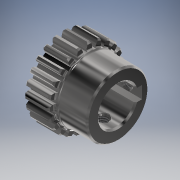
# Autodesk Inventor part: 歯車m1,z23
Saved by Autodesk Inventor 2019.2 (Build 232265000, 265)
## iProperties
Category: PARTsolutions
Company: KHK
Created: 2018-12-15
Part Number: 歯車m1,z23
Material: 鋼、高強度、低合金
Catalog Web Link: www.cadenas.de
Description: Ground Spur Gears (SSG)-
Vendor: KHK
Document SubType Name: Modeling
Designer: psadmin
Manufacturer: KHK
Mass: 4.81881 g
Surface Area: 26.6249 cm^2
Volume: 4.81881 cm^3
Density: 7.85 g/cm^3
Appearance: 鋼 - つや出し
PSOL_IDENT_0: {$CADENAS_DATA\23d-libs\khk\spur_gears\ground_spur_gears_ssg.prj},180 {VTYP=3D},{NB=SSG1-23J12},{LIN
PSOL_IDENT_1: A=SSG1-23J12},{NN=Ground Spur Gears (SSG)},{DATE=17.03.2017 04:28:20},{GEOMDATE=10.12.2014 11:17:00}
PSOL_IDENT_2: ,{VERSION=},{LINEID=18740},{WBVAR=},{WBNUMERIC=}  {NB=SSG1-23J12},{LINA=SSG1-23J12},{KT=DUMMY},{CN=S
PSOL_IDENT_3: SG1-23J12},{M=1.0},{Z=23},{A=12},{B=20},{C=23.0},{D=25.0},{E=8},{F=10},{G=18},{H=0},{I=0},{K=4},{KD=
PSOL_IDENT_4: 1.8},{M1=M4},{J=5.0},{S=S1K},{R=0.5},{N=0.5},{L=0.5},{L2=0.5},{X=3},{M11=4},{XX=4},{HIDE=0},{CBD1=0.
PSOL_IDENT_5: 0},{CBD2=0.0}
NN: Ground Spur Gears (SSG)
NB: SSG1-23J12
NBSYN: $CN.
LINA: SSG1-23J12
CN: SSG1-23J12
M: 1
Z: 23
A: 12
B: 20
C: 23
D: 25
E: 8
F: 10
G: 18
H: 0
I: 0
K: 4
KD: 1.8
M1: M4
J: 5
S: S1K
SUPPLIER: KHK
ARTICLENO: SSG1-23J12
BOMINFO: SSG1-23J12
CREATOR: CADENAS GmbH
Title: SSG1-23J12
Author: Cadenas PARTsolutions
Autodesk Inventor part; units mm, degrees
ref_plane "YZ Plane" through (0, 0, 0) normal (1, 0, 0) x (0, 1, 0)
ref_plane "XZ Plane" through (0, 0, 0) normal (0, 1, 0) x (-1, 0, 0)
ref_plane "XY Plane" through (0, 0, 0) normal (0, 0, 1) x (1, 0, 0)
sketch "Sketch_1" plane through (0, 0, 0) normal (0, 0, 1) x (1, 0, 0)
  line L0 (18, 0) -> (0, 0)
  line L1 (0, 6.5) -> (0.5, 6)
  line L2 (0.5, 6) -> (17.5, 6)
  line L3 (17.5, 6) -> (18, 6.5)
  line L4 (18, 6.5) -> (18, 9.5)
  line L5 (18, 9.5) -> (17.5, 10)
  line L6 (17.5, 10) -> (9, 10)
  arc A0 (8, 11) -> (9, 10) centre (9, 11) ccw
  line L7 (8, 11) -> (8, 12)
  line L8 (8, 12) -> (7.5, 12.5)
  line L9 (7.5, 12.5) -> (0.5, 12.5)
  line L10 (0.5, 12.5) -> (0, 12)
  line L11 (0, 12) -> (0, 6.5)
  constraints: 24 end point, 2 point on circle, 1 centre point
revolve "Revolution1" add sketch "Sketch_1" angle 360 about axis through (18, 0, 0) along (1, 0, 0)
sketch "Sketch_6" plane through (0, 0, 0) normal (1, 0, 0) x (0, 1, 0)
  line L0 (4.2, 2) -> (4.2, -2)
  line L1 (4.2, -2) -> (7.8, -2)
  line L2 (7.8, -2) -> (7.8, 2)
  line L3 (7.8, 2) -> (4.2, 2)
  constraints: 8 end point
extrude "Extrusion1" cut sketch "Sketch_6" along normal blind 20
sketch "Sketch_2" plane through (0, 0, 0) normal (0, 0, 1) x (1, 0, 0)
  line L0 (13, 0) -> (13, 12.5)
  line L1 (13, 12.5) -> (15, 12.5)
  line L2 (15, 12.5) -> (15, 10)
  line L3 (15, 10) -> (14.621, 9.621)
  line L4 (14.621, 9.621) -> (14.621, 8.179)
  line L5 (14.621, 8.179) -> (15, 7.8)
  line L6 (15, 7.8) -> (15, 0)
  line L7 (15, 0) -> (13, 0)
  line L8 (13, 0) -> (13, 12.5)
  constraints: 18 end point
revolve "Revolution2" cut sketch "Sketch_2" angle 360 about axis through (13, 0, 0) along (0, -1, 0)
thread "Thread1" size "M4x0.7" class "6H" standard "ISO Metric profile" full length
sketch "Sketch_5" plane through (0, 0, 0) normal (0, 1, 0) x (-1, 0, 0)
  line L0 (-13, 0) -> (-13, -12.5)
  line L1 (-13, -12.5) -> (-15, -12.5)
  line L2 (-15, -12.5) -> (-15, -10)
  line L3 (-15, -10) -> (-14.621, -9.621)
  line L4 (-14.621, -9.621) -> (-14.621, -6.379)
  line L5 (-14.621, -6.379) -> (-15, -6)
  line L6 (-15, -6) -> (-15, 0)
  line L7 (-15, 0) -> (-13, 0)
  line L8 (-13, 0) -> (-13, -12.5)
  constraints: 18 end point
revolve "Revolution3" cut sketch "Sketch_5" angle 360 about axis through (13, 0, 0) along (0, 0, 1)
thread "Thread2" size "M4x0.7" class "6H" standard "ISO Metric profile" full length
sketch "スケッチ5" plane through (0, 0, 0) normal (-1, 0, 0) x (0, 0, 1)
  arc A0 (0.6057, 10.9584) -> (0.5767, 10.7911) centre (1.6476, 10.6916) ccw
  arc A1 (0.7884, 11.4814) -> (0.6057, 10.9584) centre (3.4791, 10.2479) ccw
  arc A2 (1.3493, 12.427) -> (0.7884, 11.4814) centre (5.4528, 9.354) ccw
  arc A3 (-2.3733, 10.7154) -> (-2.3561, 10.5465) centre (-1.2981, 10.7397) ccw
  arc A4 (-2.3384, 11.2683) -> (-2.3733, 10.7154) centre (0.5852, 10.8065) ccw
  arc A5 (-2.0535, 12.3302) -> (-2.3384, 11.2683) centre (2.7269, 10.4783) ccw
  arc A6 (-5.1763, 9.6778) -> (-5.1141, 9.5197) centre (-4.1474, 9.9912) ccw
  arc A7 (-5.2919, 10.2196) -> (-5.1763, 9.6778) centre (-2.3521, 10.5636) ccw
  arc A8 (-5.304, 11.3189) -> (-5.2919, 10.2196) centre (-0.2013, 10.8254) ccw
  arc A9 (-7.5954, 7.9224) -> (-7.4929, 7.7869) centre (-6.6892, 8.5017) ccw
  arc A10 (-7.8529, 8.4129) -> (-7.5954, 7.9224) centre (-5.1149, 9.5373) ccw
  arc A11 (-8.1611, 9.4682) -> (-7.8529, 8.4129) centre (-3.1145, 10.3697) ccw
  arc A12 (-9.4511, 5.5794) -> (-9.3159, 5.4766) centre (-8.7349, 6.3817) ccw
  arc A13 (-9.8314, 5.9822) -> (-9.4511, 5.5794) centre (-7.4983, 7.8037) ccw
  arc A14 (-10.413, 6.9152) -> (-9.8314, 5.9822) centre (-5.7967, 9.1449) ccw
  arc A15 (-10.606, 2.8226) -> (-10.448, 2.7601) centre (-10.1328, 3.7884) ccw
  arc A16 (-11.0808, 3.1079) -> (-10.606, 2.8226) centre (-9.3257, 5.4913) ccw
  arc A17 (-11.8925, 3.8494) -> (-11.0808, 3.1079) centre (-8.049, 7.2418) ccw
  arc A18 (-10.9742, -0.1435) -> (-10.8053, -0.1611) centre (-10.7791, 0.9141) ccw
  arc A19 (-11.5084, 0.0031) -> (-10.9742, -0.1435) centre (-10.4614, 2.7716) ccw
  arc A20 (-12.4901, 0.4981) -> (-11.5084, 0.0031) centre (-9.7043, 4.8017) ccw
  arc A21 (-10.5285, -3.099) -> (-10.3611, -3.0703) centre (-10.626, -2.0279) ccw
  arc A22 (-11.0825, -3.102) -> (-10.5285, -3.099) centre (-10.8212, -0.1536) ccw
  arc A23 (-12.1613, -2.8902) -> (-11.0825, -3.102) centre (-10.6399, 2.0054) ccw
  arc A24 (-9.302, -5.8247) -> (-9.1485, -5.7519) centre (-9.6849, -4.8196) ccw
  arc A25 (-9.8346, -5.977) -> (-9.302, -5.8247) centre (-10.3785, -3.0675) ccw
  arc A26 (-10.9306, -6.0641) -> (-9.8346, -5.977) centre (-10.7864, -0.9395) ccw
  arc A27 (-7.3856, -8.1183) -> (-7.2575, -8.0068) centre (-8.0254, -7.2538) ccw
  arc A28 (-7.8574, -8.4087) -> (-7.3856, -8.1183) centre (-9.166, -5.7538) ccw
  arc A29 (-8.8892, -8.7882) -> (-7.8574, -8.4087) centre (-10.133, -3.8148) ccw
  arc A30 (-4.9214, -9.8098) -> (-4.8281, -9.6679) centre (-5.7707, -9.1501) ccw
  arc A31 (-5.2974, -10.2167) -> (-4.9214, -9.8098) centre (-7.2738, -8.0134) ccw
  arc A32 (-6.1885, -10.8606) -> (-5.2974, -10.2167) centre (-8.728, -6.4072) ccw
  arc A33 (-2.0922, -10.7738) -> (-2.0407, -10.612) centre (-3.0881, -10.3677) ccw
  arc A34 (-2.3445, -11.2671) -> (-2.0922, -10.7738) centre (-4.8421, -9.6787) ccw
  arc A35 (-3.0288, -12.1275) -> (-2.3445, -11.2671) centre (-6.6757, -8.5244) ccw
  arc A36 (0.8921, -10.9388) -> (0.8981, -10.7691) centre (-0.1764, -10.8164) ccw
  arc A37 (0.7823, -11.4818) -> (0.8921, -10.9388) centre (-2.0512, -10.6262) ccw
  arc A38 (0.3554, -12.4949) -> (0.7823, -11.4818) centre (-4.1283, -10.0094) ccw
  arc A39 (3.8103, -10.2925) -> (3.7702, -10.1274) centre (2.7483, -10.4629) ccw
  arc A40 (3.851, -10.845) -> (3.8103, -10.2925) centre (0.8917, -10.7855) ccw
  arc A41 (3.7133, -11.9357) -> (3.851, -10.845) centre (-1.2747, -10.752) ccw
  arc A42 (6.4459, -8.8828) -> (6.3628, -8.7347) centre (5.4693, -9.3334) ccw
  arc A43 (6.6342, -9.4038) -> (6.4459, -8.8828) centre (3.7686, -10.145) ccw
  arc A44 (6.7959, -10.4912) -> (6.6342, -9.4038) centre (1.6734, -10.6972) ccw
  arc A45 (8.6034, -6.8143) -> (8.4834, -6.6941) centre (7.7846, -7.5117) ccw
  arc A46 (8.9253, -7.2652) -> (8.6034, -6.8143) centre (6.3659, -8.752) ccw
  arc A47 (9.3744, -8.2687) -> (8.9253, -7.2652) centre (4.4975, -9.849) ccw
  arc A48 (10.1228, -4.2405) -> (9.9749, -4.1571) centre (9.5225, -5.1329) ccw
  arc A49 (10.5544, -4.5878) -> (10.1228, -4.2405) centre (8.4911, -6.71) ccw
  arc A50 (11.2576, -5.4329) -> (10.5544, -4.5878) centre (6.9879, -8.2704) ccw
  arc A51 (10.8915, -1.3521) -> (10.7266, -1.3118) centre (10.5542, -2.3734) ccw
  arc A52 (11.4008, -1.5701) -> (10.8915, -1.3521) centre (9.9866, -4.1703) ccw
  arc A53 (12.3059, -2.1942) -> (11.4008, -1.5701) centre (8.9601, -6.0784) ccw
  arc A54 (10.8524, 1.6365) -> (10.6827, 1.6309) centre (10.8032, 0.5621) ccw
  arc A55 (11.4017, 1.564) -> (10.8524, 1.6365) centre (10.7414, -1.3213) ccw
  arc A56 (12.4416, 1.2073) -> (11.4017, 1.564) centre (10.2678, -3.4356) ccw
  arc A57 (10.0085, 4.5038) -> (9.8465, 4.4526) centre (10.2509, 3.456) ccw
  arc A58 (10.5569, 4.5821) -> (10.0085, 4.5038) centre (10.6995, 1.6257) ccw
  arc A59 (11.6545, 4.5192) -> (10.5569, 4.5821) centre (10.8139, -0.538) ccw
  arc A60 (8.4222, 7.037) -> (8.2801, 6.944) centre (8.9384, 6.0935) ccw
  arc A61 (8.9292, 7.2604) -> (8.4222, 7.037) centre (9.8642, 4.4521) ccw
  arc A62 (10.003, 7.496) -> (8.9292, 7.2604) centre (10.558, 2.3995) ccw
  arc A63 (6.2113, 9.0484) -> (6.0996, 8.9205) centre (6.9629, 8.279) ccw
  arc A64 (6.6392, 9.4003) -> (6.2113, 9.0484) centre (8.2972, 6.9483) ccw
  arc A65 (7.6097, 9.9168) -> (6.6392, 9.4003) centre (9.5191, 5.1591) ccw
  arc A66 (3.5398, 10.3886) -> (3.4667, 10.2353) centre (4.4711, 9.8506) ccw
  arc A67 (3.8568, 10.8429) -> (3.5398, 10.3886) centre (6.1149, 8.9292) ccw
  arc A68 (4.652, 11.6021) -> (3.8568, 10.8429) centre (7.7742, 7.536) ccw
  arc A69 (-0.5767, 10.7911) -> (-0.6057, 10.9584) centre (-1.6476, 10.6916) ccw
  arc A70 (-0.6057, 10.9584) -> (-0.7884, 11.4814) centre (-3.4791, 10.2479) ccw
  arc A71 (-0.7884, 11.4814) -> (-1.3493, 12.427) centre (-5.4528, 9.354) ccw
  arc A72 (-3.4667, 10.2353) -> (-3.5398, 10.3886) centre (-4.4711, 9.8506) ccw
  arc A73 (-3.5398, 10.3886) -> (-3.8568, 10.8429) centre (-6.1149, 8.9292) ccw
  arc A74 (-3.8568, 10.8429) -> (-4.652, 11.6021) centre (-7.7742, 7.536) ccw
  arc A75 (-6.0996, 8.9205) -> (-6.2113, 9.0484) centre (-6.9629, 8.279) ccw
  arc A76 (-6.2113, 9.0484) -> (-6.6392, 9.4003) centre (-8.2972, 6.9483) ccw
  arc A77 (-6.6392, 9.4003) -> (-7.6097, 9.9168) centre (-9.5191, 5.1591) ccw
  arc A78 (-8.2801, 6.944) -> (-8.4222, 7.037) centre (-8.9384, 6.0935) ccw
  arc A79 (-8.4222, 7.037) -> (-8.9292, 7.2604) centre (-9.8642, 4.4521) ccw
  arc A80 (-8.9292, 7.2604) -> (-10.003, 7.496) centre (-10.558, 2.3995) ccw
  arc A81 (-9.8465, 4.4526) -> (-10.0085, 4.5038) centre (-10.2509, 3.456) ccw
  arc A82 (-10.0085, 4.5038) -> (-10.5569, 4.5821) centre (-10.6995, 1.6257) ccw
  arc A83 (-10.5569, 4.5821) -> (-11.6545, 4.5192) centre (-10.8139, -0.538) ccw
  arc A84 (-10.6827, 1.6309) -> (-10.8524, 1.6365) centre (-10.8032, 0.5621) ccw
  arc A85 (-10.8524, 1.6365) -> (-11.4017, 1.564) centre (-10.7414, -1.3213) ccw
  arc A86 (-11.4017, 1.564) -> (-12.4416, 1.2073) centre (-10.2678, -3.4356) ccw
  arc A87 (-10.7266, -1.3118) -> (-10.8915, -1.3521) centre (-10.5542, -2.3734) ccw
  arc A88 (-10.8915, -1.3521) -> (-11.4008, -1.5701) centre (-9.9866, -4.1703) ccw
  arc A89 (-11.4008, -1.5701) -> (-12.3059, -2.1942) centre (-8.9601, -6.0784) ccw
  arc A90 (-9.9749, -4.1571) -> (-10.1228, -4.2405) centre (-9.5225, -5.1329) ccw
  arc A91 (-10.1228, -4.2405) -> (-10.5544, -4.5878) centre (-8.4911, -6.71) ccw
  arc A92 (-10.5544, -4.5878) -> (-11.2576, -5.4329) centre (-6.9879, -8.2704) ccw
  arc A93 (-8.4834, -6.6941) -> (-8.6034, -6.8143) centre (-7.7846, -7.5117) ccw
  arc A94 (-8.6034, -6.8143) -> (-8.9253, -7.2652) centre (-6.3659, -8.752) ccw
  arc A95 (-8.9253, -7.2652) -> (-9.3744, -8.2687) centre (-4.4975, -9.849) ccw
  arc A96 (-6.3628, -8.7347) -> (-6.4459, -8.8828) centre (-5.4693, -9.3334) ccw
  arc A97 (-6.4459, -8.8828) -> (-6.6342, -9.4038) centre (-3.7686, -10.145) ccw
  arc A98 (-6.6342, -9.4038) -> (-6.7959, -10.4912) centre (-1.6734, -10.6972) ccw
  arc A99 (-3.7702, -10.1274) -> (-3.8103, -10.2925) centre (-2.7483, -10.4629) ccw
  arc A100 (-3.8103, -10.2925) -> (-3.851, -10.845) centre (-0.8917, -10.7855) ccw
  arc A101 (-3.851, -10.845) -> (-3.7133, -11.9357) centre (1.2747, -10.752) ccw
  arc A102 (-0.8981, -10.7691) -> (-0.8921, -10.9388) centre (0.1764, -10.8164) ccw
  arc A103 (-0.8921, -10.9388) -> (-0.7823, -11.4818) centre (2.0512, -10.6262) ccw
  arc A104 (-0.7823, -11.4818) -> (-0.3554, -12.4949) centre (4.1283, -10.0094) ccw
  arc A105 (2.0407, -10.612) -> (2.0922, -10.7738) centre (3.0881, -10.3677) ccw
  arc A106 (2.0922, -10.7738) -> (2.3445, -11.2671) centre (4.8421, -9.6787) ccw
  arc A107 (2.3445, -11.2671) -> (3.0288, -12.1275) centre (6.6757, -8.5244) ccw
  arc A108 (4.8281, -9.6679) -> (4.9214, -9.8098) centre (5.7707, -9.1501) ccw
  arc A109 (4.9214, -9.8098) -> (5.2974, -10.2167) centre (7.2738, -8.0134) ccw
  arc A110 (5.2974, -10.2167) -> (6.1885, -10.8606) centre (8.728, -6.4072) ccw
  arc A111 (7.2575, -8.0068) -> (7.3856, -8.1183) centre (8.0254, -7.2538) ccw
  arc A112 (7.3856, -8.1183) -> (7.8574, -8.4087) centre (9.166, -5.7538) ccw
  arc A113 (7.8574, -8.4087) -> (8.8892, -8.7882) centre (10.133, -3.8148) ccw
  arc A114 (9.1485, -5.7519) -> (9.302, -5.8247) centre (9.6849, -4.8196) ccw
  arc A115 (9.302, -5.8247) -> (9.8346, -5.977) centre (10.3785, -3.0675) ccw
  arc A116 (9.8346, -5.977) -> (10.9306, -6.0641) centre (10.7864, -0.9395) ccw
  arc A117 (10.3611, -3.0703) -> (10.5285, -3.099) centre (10.626, -2.0279) ccw
  arc A118 (10.5285, -3.099) -> (11.0825, -3.102) centre (10.8212, -0.1536) ccw
  arc A119 (11.0825, -3.102) -> (12.1613, -2.8902) centre (10.6399, 2.0054) ccw
  arc A120 (10.8053, -0.1611) -> (10.9742, -0.1435) centre (10.7791, 0.9141) ccw
  arc A121 (10.9742, -0.1435) -> (11.5084, 0.0031) centre (10.4614, 2.7716) ccw
  arc A122 (11.5084, 0.0031) -> (12.4901, 0.4981) centre (9.7043, 4.8017) ccw
  arc A123 (10.448, 2.7601) -> (10.606, 2.8226) centre (10.1328, 3.7884) ccw
  arc A124 (10.606, 2.8226) -> (11.0808, 3.1079) centre (9.3257, 5.4913) ccw
  arc A125 (11.0808, 3.1079) -> (11.8925, 3.8494) centre (8.049, 7.2418) ccw
  arc A126 (9.3159, 5.4766) -> (9.4511, 5.5794) centre (8.7349, 6.3817) ccw
  arc A127 (9.4511, 5.5794) -> (9.8314, 5.9822) centre (7.4983, 7.8037) ccw
  arc A128 (9.8314, 5.9822) -> (10.413, 6.9152) centre (5.7967, 9.1449) ccw
  arc A129 (7.4929, 7.7869) -> (7.5954, 7.9224) centre (6.6892, 8.5017) ccw
  arc A130 (7.5954, 7.9224) -> (7.8529, 8.4129) centre (5.1149, 9.5373) ccw
  arc A131 (7.8529, 8.4129) -> (8.1611, 9.4682) centre (3.1145, 10.3697) ccw
  arc A132 (5.1141, 9.5197) -> (5.1763, 9.6778) centre (4.1474, 9.9912) ccw
  arc A133 (5.1763, 9.6778) -> (5.2919, 10.2196) centre (2.3521, 10.5636) ccw
  arc A134 (5.2919, 10.2196) -> (5.304, 11.3189) centre (0.2013, 10.8254) ccw
  arc A135 (2.3561, 10.5465) -> (2.3733, 10.7154) centre (1.2981, 10.7397) ccw
  arc A136 (2.3733, 10.7154) -> (2.3384, 11.2683) centre (-0.5852, 10.8065) ccw
  arc A137 (2.3384, 11.2683) -> (2.0535, 12.3302) centre (-2.7269, 10.4783) ccw
  arc A138 (0.547, 10.2354) -> (-0.547, 10.2354) centre (0, 0) ccw
  arc A139 (-2.2348, 10.0034) -> (-3.2882, 9.7083) centre (0, 0) ccw
  arc A140 (-4.8508, 9.0295) -> (-5.7855, 8.4611) centre (0, 0) ccw
  arc A141 (-7.107, 7.386) -> (-7.8537, 6.5864) centre (0, 0) ccw
  arc A142 (-8.8362, 5.1946) -> (-9.3395, 4.2233) centre (0, 0) ccw
  arc A143 (-9.91, 2.618) -> (-10.1326, 1.5469) centre (0, 0) ccw
  arc A144 (-10.2489, -0.1528) -> (-10.1742, -1.2442) centre (0, 0) ccw
  arc A145 (-9.8276, -2.9122) -> (-9.4612, -3.943) centre (0, 0) ccw
  arc A146 (-8.6775, -5.4557) -> (-8.0466, -6.3494) centre (0, 0) ccw
  arc A147 (-6.8837, -7.5945) -> (-6.0351, -8.2849) centre (0, 0) ccw
  arc A148 (-4.5795, -9.1701) -> (-3.5761, -9.6059) centre (0, 0) ccw
  arc A149 (-1.9356, -10.0656) -> (-0.8518, -10.2145) centre (0, 0) ccw
  arc A150 (0.8518, -10.2145) -> (1.9356, -10.0656) centre (0, 0) ccw
  arc A151 (3.5761, -9.6059) -> (4.5795, -9.1701) centre (0, 0) ccw
  arc A152 (6.0351, -8.2849) -> (6.8837, -7.5945) centre (0, 0) ccw
  arc A153 (8.0466, -6.3494) -> (8.6775, -5.4557) centre (0, 0) ccw
  arc A154 (9.4612, -3.943) -> (9.8276, -2.9122) centre (0, 0) ccw
  arc A155 (10.1742, -1.2442) -> (10.2489, -0.1528) centre (0, 0) ccw
  arc A156 (10.1326, 1.5469) -> (9.91, 2.618) centre (0, 0) ccw
  arc A157 (9.3395, 4.2233) -> (8.8362, 5.1946) centre (0, 0) ccw
  arc A158 (7.8537, 6.5864) -> (7.107, 7.386) centre (0, 0) ccw
  arc A159 (5.7855, 8.4611) -> (4.8508, 9.0295) centre (0, 0) ccw
  arc A160 (3.2882, 9.7083) -> (2.2348, 10.0034) centre (0, 0) ccw
  arc A161 (-1.3493, 12.427) -> (-2.0535, 12.3302) centre (0, 0) ccw
  arc A162 (-4.652, 11.6021) -> (-5.304, 11.3189) centre (0, 0) ccw
  arc A163 (-7.6097, 9.9168) -> (-8.1611, 9.4682) centre (0, 0) ccw
  arc A164 (-10.003, 7.496) -> (-10.413, 6.9152) centre (0, 0) ccw
  arc A165 (-11.6545, 4.5192) -> (-11.8925, 3.8494) centre (0, 0) ccw
  arc A166 (-12.4416, 1.2073) -> (-12.4901, 0.4981) centre (0, 0) ccw
  arc A167 (-12.3059, -2.1942) -> (-12.1613, -2.8902) centre (0, 0) ccw
  arc A168 (-11.2576, -5.4329) -> (-10.9306, -6.0641) centre (0, 0) ccw
  arc A169 (-9.3744, -8.2687) -> (-8.8892, -8.7882) centre (0, 0) ccw
  arc A170 (-6.7959, -10.4912) -> (-6.1885, -10.8606) centre (0, 0) ccw
  arc A171 (-3.7133, -11.9357) -> (-3.0288, -12.1275) centre (0, 0) ccw
  arc A172 (-0.3554, -12.4949) -> (0.3554, -12.4949) centre (0, 0) ccw
  arc A173 (3.0288, -12.1275) -> (3.7133, -11.9357) centre (0, 0) ccw
  arc A174 (6.1885, -10.8606) -> (6.7959, -10.4912) centre (0, 0) ccw
  arc A175 (8.8892, -8.7882) -> (9.3744, -8.2687) centre (0, 0) ccw
  arc A176 (10.9306, -6.0641) -> (11.2576, -5.4329) centre (0, 0) ccw
  arc A177 (12.1613, -2.8902) -> (12.3059, -2.1942) centre (0, 0) ccw
  arc A178 (12.4901, 0.4981) -> (12.4416, 1.2073) centre (0, 0) ccw
  arc A179 (11.8925, 3.8494) -> (11.6545, 4.5192) centre (0, 0) ccw
  arc A180 (10.413, 6.9152) -> (10.003, 7.496) centre (0, 0) ccw
  arc A181 (8.1611, 9.4682) -> (7.6097, 9.9168) centre (0, 0) ccw
  arc A182 (5.304, 11.3189) -> (4.652, 11.6021) centre (0, 0) ccw
  arc A183 (2.0535, 12.3302) -> (1.3493, 12.427) centre (0, 0) ccw
  line L0 (0.547, 10.2354) -> (0.5767, 10.7911)
  line L1 (-2.2348, 10.0034) -> (-2.3561, 10.5465)
  line L2 (-4.8508, 9.0295) -> (-5.1141, 9.5197)
  line L3 (-7.107, 7.386) -> (-7.4929, 7.7869)
  line L4 (-8.8362, 5.1946) -> (-9.3159, 5.4766)
  line L5 (-9.91, 2.618) -> (-10.448, 2.7601)
  line L6 (-10.2489, -0.1528) -> (-10.8053, -0.1611)
  line L7 (-9.8276, -2.9122) -> (-10.3611, -3.0703)
  line L8 (-8.6775, -5.4557) -> (-9.1485, -5.7519)
  line L9 (-6.8837, -7.5945) -> (-7.2575, -8.0068)
  line L10 (-4.5795, -9.1701) -> (-4.8281, -9.6679)
  line L11 (-1.9356, -10.0656) -> (-2.0407, -10.612)
  line L12 (0.8518, -10.2145) -> (0.8981, -10.7691)
  line L13 (3.5761, -9.6059) -> (3.7702, -10.1274)
  line L14 (6.0351, -8.2849) -> (6.3628, -8.7347)
  line L15 (8.0466, -6.3494) -> (8.4834, -6.6941)
  line L16 (9.4612, -3.943) -> (9.9749, -4.1571)
  line L17 (10.1742, -1.2442) -> (10.7266, -1.3118)
  line L18 (10.1326, 1.5469) -> (10.6827, 1.6309)
  line L19 (9.3395, 4.2233) -> (9.8465, 4.4526)
  line L20 (7.8537, 6.5864) -> (8.2801, 6.944)
  line L21 (5.7855, 8.4611) -> (6.0996, 8.9205)
  line L22 (3.2882, 9.7083) -> (3.4667, 10.2353)
  line L23 (-0.547, 10.2354) -> (-0.5767, 10.7911)
  line L24 (-3.2882, 9.7083) -> (-3.4667, 10.2353)
  line L25 (-5.7855, 8.4611) -> (-6.0996, 8.9205)
  line L26 (-7.8537, 6.5864) -> (-8.2801, 6.944)
  line L27 (-9.3395, 4.2233) -> (-9.8465, 4.4526)
  line L28 (-10.1326, 1.5469) -> (-10.6827, 1.6309)
  line L29 (-10.1742, -1.2442) -> (-10.7266, -1.3118)
  line L30 (-9.4612, -3.943) -> (-9.9749, -4.1571)
  line L31 (-8.0466, -6.3494) -> (-8.4834, -6.6941)
  line L32 (-6.0351, -8.2849) -> (-6.3628, -8.7347)
  line L33 (-3.5761, -9.6059) -> (-3.7702, -10.1274)
  line L34 (-0.8518, -10.2145) -> (-0.8981, -10.7691)
  line L35 (1.9356, -10.0656) -> (2.0407, -10.612)
  line L36 (4.5795, -9.1701) -> (4.8281, -9.6679)
  line L37 (6.8837, -7.5945) -> (7.2575, -8.0068)
  line L38 (8.6775, -5.4557) -> (9.1485, -5.7519)
  line L39 (9.8276, -2.9122) -> (10.3611, -3.0703)
  line L40 (10.2489, -0.1528) -> (10.8053, -0.1611)
  line L41 (9.91, 2.618) -> (10.448, 2.7601)
  line L42 (8.8362, 5.1946) -> (9.3159, 5.4766)
  line L43 (7.107, 7.386) -> (7.4929, 7.7869)
  line L44 (4.8508, 9.0295) -> (5.1141, 9.5197)
  line L45 (2.2348, 10.0034) -> (2.3561, 10.5465)
  line L46 (-14.5, 0) -> (14.5, 0)
  line L47 (0, -14.5) -> (0, 14.5)
  line L48 (32.5, 12.5) -> (102.5, 12.5)
  line L49 (32.5, 4.5) -> (102.5, 4.5)
  line L50 (32.5, -3.5) -> (102.5, -3.5)
  line L51 (32.5, -11.5) -> (102.5, -11.5)
  line L52 (32.5, -19.5) -> (102.5, -19.5)
  line L53 (32.5, -27.5) -> (102.5, -27.5)
  line L54 (32.5, -35.5) -> (102.5, -35.5)
  line L55 (32.5, -43.5) -> (102.5, -43.5)
  line L56 (32.5, -51.5) -> (102.5, -51.5)
  line L57 (32.5, -59.5) -> (102.5, -59.5)
  line L58 (32.5, -67.5) -> (102.5, -67.5)
  line L59 (32.5, -75.5) -> (102.5, -75.5)
  line L60 (32.5, -83.5) -> (102.5, -83.5)
  line L61 (32.5, 12.5) -> (32.5, -83.5)
  line L62 (102.5, 12.5) -> (102.5, -83.5)
  line L63 (67.5, 4.5) -> (67.5, -83.5)
  circle A184 centre (0, 0) radius 12.5 projected
  point P0 (38.5, 6.5)
  point P1 (41, -1.5)
  point P2 (41, -9.5)
  point P3 (38.5, -17.5)
  point P4 (41, -25.5)
  point P5 (36, -33.5)
  point P6 (38.5, -41.5)
  point P7 (38.5, -49.5)
  point P8 (38.5, -57.5)
  point P9 (41, -65.5)
  point P10 (41, -73.5)
  point P11 (38.5, -81.5)
  point P12 (68.5, -1.5)
  point P13 (83.5, -9.5)
  point P14 (84.75, -17.5)
  point P15 (81, -25.5)
  point P16 (83.5, -33.5)
  point P17 (77.25, -41.5)
  point P18 (83.5, -49.5)
  point P19 (81, -57.5)
  point P20 (78.5, -65.5)
  point P21 (1, 28)
  point P22 (1, 22)
  point P23 (18.25, 28)
  point P24 (20.375, 22)
  constraints: 276 point on circle, 138 centre point, 124 end point, 2 horizontal alignment, 2 midpoint, 190 other
extrude "押し出し2" cut sketch "スケッチ5" against normal blind 10 contours A0 L0 A138 L47 A184 A2 A1 | A138 L23 A69 A70 A71 A184 L47 | A184 A68 A67 A66 L22 A160 L45 A135 A136 A137 | L46 A184 A20 A19 | A19 A18 L6 A144 L29 A87 A88 A89 A184 L46 | L46 A184 A53 A52 A51 L17 A155 L40 A120 A121 | A121 A122 A184 L46 | A184 A65 A64 A63 L21 A159 L44 A132 A133 A134 | A5 A4 A3 L1 A139 L24 A72 A73 A74 A184 | A184 A35 A34 A33 L11 A149 L34 A102 A103 A104 | A38 A37 A36 L12 A150 L35 A105 A106 A107 A184 | A184 A62 A61 A60 L20 A158 L43 A129 A130 A131 | A8 A7 A6 L2 A140 L25 A75 A76 A77 A184 | A184 A17 A16 A15 L5 A143 L28 A84 A85 A86 | A23 A22 A21 L7 A145 L30 A90 A91 A92 A184 | A56 A55 A54 L18 A156 L41 A123 A124 A125 A184 | A184 A50 A49 A48 L16 A154 L39 A117 A118 A119 | A184 A32 A31 A30 L10 A148 L33 A99 A100 A101 | A41 A40 A39 L13 A151 L36 A108 A109 A110 A184 | A184 A59 A58 A57 L19 A157 L42 A126 A127 A128 | A11 A10 A9 L3 A141 L26 A78 A79 A80 A184 | A184 A14 A13 A12 L4 A142 L27 A81 A82 A83 | A26 A25 A24 L8 A146 L31 A93 A94 A95 A184 | A184 A47 A46 A45 L15 A153 L38 A114 A115 A116 | A184 A29 A28 A27 L9 A147 L32 A96 A97 A98 | A44 A43 A42 L14 A152 L37 A111 A112 A113 A184
body "Solid1"
